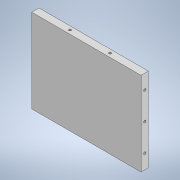
# Autodesk Inventor part: front
Saved by Autodesk Inventor 2022.2 (Build 262287030, 287C)
## iProperties
Created: 2022-01-28
Part Number: front
Material: Generic
Document SubType Name: Modeling
Designer: Tapendra
Density: 1 g/cm^3
Appearance: Default
Author: Tapendra
Autodesk Inventor part; units mm, degrees
ref_plane "YZ Plane" through (0, 0, 0) normal (1, 0, 0) x (0, 1, 0)
ref_plane "XZ Plane" through (0, 0, 0) normal (0, 1, 0) x (-1, 0, 0)
ref_plane "XY Plane" through (0, 0, 0) normal (0, 0, 1) x (1, 0, 0)
sketch "Sketch1" plane through (0, 0, 0) normal (0, 0, 1) x (1, 0, 0)
  line L0 (-75, 57.5) -> (75, 57.5)
  line L1 (75, 57.5) -> (75, -57.5)
  line L2 (75, -57.5) -> (-75, -57.5)
  line L3 (-75, -57.5) -> (-75, 57.5)
  line L4 (-75, 57.5) -> (75, -57.5) construction
  line L5 (75, 57.5) -> (-75, -57.5) construction
  point P0 (0, 0)
  dimension "d0" = 150
  dimension "d1" = 115
  constraints: 12 end point, 2 midpoint, 2 parallel, 1 horizontal, 1 perpendicular
  measures "d0" distance of L0.start L0.end
  measures "d1" distance of L0.end L1.end
extrude "Extrusion1" add sketch "Sketch1" along normal mid plane 10
sketch "Sketch2" plane through (75, -57.5, 5) normal (1, 0, 0) x (0, 0, -1)
  line L0 (10, 0) -> (0, 0) projected
  line L1 (0, 0) -> (0, 115) projected
  point P0 (5, 57.5)
  point P1 (5, 20)
  point P2 (5, 57.5)
  point P3 (5, 95)
  dimension "d4" = 20
  dimension "d5" = 5
  dimension "d8" = 37.5
  constraints: 1 vertical, 2 other
  measures "d4" distance from line of L0 point (5, 20)
  measures "d5" distance from line of L1 point (5, 20)
  measures "d8" distance of point (5, 20) point (5, 57.5)
hole "Hole1" at (75, -37.5, 0) at (75, 0, 0) at (75, 37.5, 0) direction (-1, 0, 0) diameter 3.175 depth 5
sketch "Sketch3" plane through (-75, 57.5, 5) normal (0, 1, 0) x (1, 0, 0)
  line L0 (150, 10) -> (150, 0) projected
  line L1 (0, 10) -> (150, 10) projected
  point P0 (75, 5)
  point P1 (102.5, 5)
  point P2 (47.5, 5)
  dimension "d20" = 47.5
  dimension "d21" = 5
  dimension "d24" = 55
  constraints: 1 horizontal, 1 other
  measures "d20" distance from line of L0 point (102.5, 5)
  measures "d21" distance from line of L1 point (102.5, 5)
  measures "d24" distance of point (102.5, 5) point (47.5, 5)
hole "Hole2" at (27.5, 57.5, 0) at (-27.5, 57.5, 0) direction (0, -1, 0) diameter 3.175 depth 5
sketch "Sketch4" plane through (-75, -57.5, 5) normal (0, -1, 0) x (1, 0, 0)
  line L0 (150, -10) -> (150, 0) projected
  line L1 (0, 0) -> (150, 0) projected
  point P0 (75, -5)
  point P1 (102.5, -5)
  point P2 (47.5, -5)
  dimension "d36" = 47.5
  dimension "d37" = 5
  dimension "d40" = 55
  constraints: 1 horizontal, 1 other
  measures "d36" distance from line of L0 point (102.5, -5)
  measures "d37" distance from line of L1 point (102.5, -5)
  measures "d40" distance of point (102.5, -5) point (47.5, -5)
hole "Hole3" at (27.5, -57.5, 0) at (-27.5, -57.5, 0) direction (0, 1, 0) diameter 3.175 depth 5
sketch "Sketch5" plane through (-75, -57.5, 5) normal (-1, 0, 0) x (0, 0, 1)
  line L0 (0, 0) -> (-10, 0) projected
  line L1 (-10, 0) -> (-10, 115) projected
  point P0 (-5, 57.5)
  point P1 (-5, 20)
  point P2 (-5, 57.5)
  point P3 (-5, 95)
  dimension "d52" = 20
  dimension "d53" = 5
  dimension "d56" = 37.5
  constraints: 1 vertical, 2 other
  measures "d52" distance from line of L0 point (-5, 20)
  measures "d53" distance from line of L1 point (-5, 20)
  measures "d56" distance of point (-5, 20) point (-5, 57.5)
hole "Hole4" at (-75, -37.5, 0) at (-75, 0, 0) at (-75, 37.5, 0) direction (1, 0, 0) diameter 3.175 depth 5
body "Solid1"
